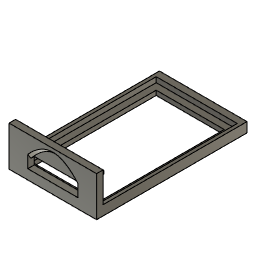
sdr2 (Autodesk Fusion 360 design; units mm, degrees)
Autodesk Fusion 360 part; units mm, degrees
sketch "Sketch1" plane through (0, 0, 0) normal (0, 1, 0) x (1, 0, 0)
  line L0 (0, 0) -> (15, 0)
  line L1 (15, 0) -> (15, -1.85)
  line L2 (15, -1.85) -> (0, -1.85)
  line L3 (0, -1.85) -> (0, 0)
  line L4 (-0.2, -2.05) -> (15.2, -2.05)
  line L5 (15.2, -2.05) -> (15.2, 0.2)
  line L6 (15.2, 0.2) -> (-0.2, 0.2)
  line L7 (-0.2, 0.2) -> (-0.2, -2.05)
  spline S0 degree 5 poles (-0.2, -2.05) (0.108, -2.4292) (0.724, -3.1546) (1.648, -4.1433) (2.88, -5.2595) (4.42, -6.2953) (5.96, -6.9394) (7.5, -7.16) (9.04, -6.9394) (10.58, -6.2953) (12.12, -5.2595) (13.352, -4.1433) (14.276, -3.1546) (14.892, -2.4292) (15.2, -2.05) knots 0 0 0 0 0 0 0.1 0.2 0.3 0.4 0.5 0.6 0.7 0.8 0.9 1 1 1 1 1 1
  line L8 (-6.2, -9.05) -> (21.2, -9.05)
  line L9 (21.2, -9.05) -> (21.2, 3.2)
  line L10 (21.2, 3.2) -> (-6.2, 3.2)
  line L11 (-6.2, 3.2) -> (-6.2, -9.05)
  line L12 (-4.95, 0.2) -> (19.95, 0.2)
  line L13 (19.95, 0.2) -> (19.95, 1.8)
  line L14 (19.95, 1.8) -> (-4.95, 1.8)
  line L15 (-4.95, 1.8) -> (-4.95, 0.2)
  line L16 (-4.95, 0.2) -> (-5.95, 0.2)
  line L17 (-5.95, 0.2) -> (-5.95, 3.2)
  line L18 (-5.95, 3.2) -> (-4.95, 3.2)
  line L19 (-4.95, 3.2) -> (-4.95, 0.2)
  line L20 (19.95, 0.2) -> (20.95, 0.2)
  line L21 (20.95, 0.2) -> (20.95, 3.2)
  line L22 (20.95, 3.2) -> (19.95, 3.2)
  line L23 (19.95, 3.2) -> (19.95, 0.2)
  point P0 (7.5, -7.05)
  dimension "d1" = 15
  dimension "d2" = 1.85
  dimension "d3" = 0.2
  dimension "d4" = 0.2
  dimension "d5" = 0.2
  dimension "d6" = 0.2
  dimension "d8" = 5
  dimension "d9" = 3
  dimension "d10" = 6
  dimension "d11" = 6
  dimension "d12" = 7
  dimension "d13" = 24.9
  dimension "d14" = 1.6
  dimension "d15" = 4.75
  dimension "d24" = 1
  dimension "d25" = 1
  dimension "d26" = 3
  constraint horizontal L0
  constraint vertical L1
  constraint horizontal L2
  constraint vertical L3
  constraint coincident L0.start L3.end
  constraint horizontal L4
  constraint vertical L5
  constraint horizontal L6
  constraint vertical L7
  constraint horizontal L8
  constraint vertical L9
  constraint horizontal L10
  constraint vertical L11
  constraint horizontal L12
  constraint vertical L13
  constraint horizontal L14
  constraint vertical L15
  constraint horizontal L16
  constraint vertical L17
  constraint horizontal L18
  constraint vertical L19
  constraint horizontal L20
  constraint vertical L21
  constraint horizontal L22
  constraint vertical L23
  measures "d1" distance of L0.start L0.end
  measures "d2" distance of L0.start L2.end
  measures "d3" distance of L3 L7
  measures "d4" distance of L2 L4
  measures "d5" distance of L1 L5
  measures "d6" distance of L0 L6
  measures "d8" distance of L4 P0
  measures "d9" distance of L6 L10
  measures "d10" distance of L7 L11
  measures "d11" distance of L5 L9
  measures "d12" distance of L4 L8
  measures "d13" distance of L12.start L12.end
  measures "d14" distance of L12.start L14.end
  measures "d15" distance of L7 L15
  measures "d24" distance of L12.start L16.end
  measures "d25" distance of L12.end L20.end
  measures "d26" distance of L12.end L22.end
extrude "Extrude1" add sketch "Sketch1" against normal blind 2 contours L5 L7 S0 L8 L9 L10 L11 L12 L16 L17 L20 L21 | L10 L15 L16 L17 L18 L19 | L10 L13 L20 L21 L22 L23 | L10 L14 L19 L23
extrude "Extrude2" add sketch "Sketch1" against normal blind 1 contours L4 S0
chamfer "Chamfer1" distance 1 angle 45 1 edges at (7.5, -1, 2.05)
chamfer "Chamfer2" distance 1 angle 45 1 edges at (7.5, -2, 7.05)
extrude "Extrude3" add sketch "Sketch1" against normal blind 2 contours L6 L12 L13 L14 L15 L19 L23
extrude "Extrude4" add sketch "Sketch1" along normal blind 42.2 contours L10 L15 L16 L17 L18 L19 | L10 L13 L20 L21 L22 L23 | L10 L14 L19 L23
sketch "Sketch2" plane through (0, 42.2, 0) normal (0, 1, 0) x (-1, 0, 0)
  line L0 (-19.95, -0.2) -> (-20.95, -0.2)
  line L1 (-20.95, -0.2) -> (-20.95, -3.2)
  line L2 (-20.95, -3.2) -> (5.95, -3.2)
  line L3 (5.95, -3.2) -> (5.95, -0.2)
  line L4 (5.95, -0.2) -> (4.95, -0.2)
  line L5 (4.95, -0.2) -> (4.95, -1.8)
  line L6 (4.95, -1.8) -> (-19.95, -1.8)
  line L7 (-19.95, -1.8) -> (-19.95, -0.2)
  line L8 (-20.95, -0.2) -> (5.95, -0.2)
  line L9 (5.95, -0.2) -> (5.95, -3.2)
  line L10 (5.95, -3.2) -> (-20.95, -3.2)
  line L11 (-20.95, -3.2) -> (-20.95, -0.2)
  constraint horizontal L8
  constraint vertical L9
  constraint horizontal L10
  constraint vertical L11
  constraint coincident L2.end L3.start
  constraint coincident L0.end L1.start
extrude "Extrude5" add sketch "Sketch2" along normal blind 2
sketch "Sketch3" plane through (0, 0, -1.8) normal (0, 0, 1) x (-1, 0, 0)
  line L0 (4.95, 0) -> (-19.95, 0)
  line L1 (-19.95, 0) -> (-19.95, -42.2)
  line L2 (-19.95, -42.2) -> (4.95, -42.2)
  line L3 (4.95, -42.2) -> (4.95, 0)
  line L4 (2.95, -2) -> (-17.95, -2)
  line L5 (-17.95, -2) -> (-17.95, -40.2)
  line L6 (-17.95, -40.2) -> (2.95, -40.2)
  line L7 (2.95, -40.2) -> (2.95, -2)
  line L8 (6.2, 0) -> (-21.2, 0)
  dimension "d31" = 2
  dimension "d32" = 2
  dimension "d33" = 2
  dimension "d34" = 2
  constraint horizontal L4
  constraint vertical L5
  constraint horizontal L6
  constraint vertical L7
  measures "d31" distance of L2 L6
  measures "d32" distance of L1 L5
  measures "d33" distance of L4 L8
  measures "d34" distance of L3 L7
extrude "Extrude6" cut sketch "Sketch3" against normal blind 3 contours L4 L5 L6 L7
extrude "Extrude7" cut 1 faces at (-6.2, -0.6667, 0.8833) along direction (1, 0, 0) blind 0.25
extrude "Extrude8" cut 1 faces at (21.2, -0.6667, 4.9667) along direction (-1, 0, 0) blind 0.25
sketch "Sketch4" plane through (0, 0, 0) normal (0, 1, 0) x (-1, 0, 0)
  line L0 (-20.95, 9.05) -> (-20.95, -0.2)
  line L1 (-20.95, -0.2) -> (-19.95, -0.2)
  line L2 (-19.95, -0.2) -> (-19.95, -1.8)
  line L3 (-19.95, -1.8) -> (4.95, -1.8)
  line L4 (4.95, -1.8) -> (4.95, -0.2)
  line L5 (4.95, -0.2) -> (5.95, -0.2)
  line L6 (5.95, -0.2) -> (5.95, 9.05)
  line L7 (5.95, 9.05) -> (-20.95, 9.05)
  line L8 (-15.2, -0.2) -> (-15.2, 2.05)
  line L9 (-15.2, 2.05) -> (0.2, 2.05)
  line L10 (0.2, 2.05) -> (0.2, -0.2)
  line L11 (0.2, -0.2) -> (-15.2, -0.2)
  line L12 (-15.2, 2.05) -> (0.2, 2.05)
  line L13 (0.2, 2.05) -> (0.2, 6.05)
  line L14 (0.2, 6.05) -> (-15.2, 6.05)
  line L15 (-15.2, 6.05) -> (-15.2, 2.05)
  dimension "d41" = 15.4
  dimension "d42" = 4
  constraint horizontal L12
  constraint vertical L13
  constraint horizontal L14
  constraint vertical L15
  constraint coincident L8.end L9.start
  measures "d41" distance of L8.end L9.end
  measures "d42" distance of L8.end L14.end
extrude "Extrude9" add sketch "Sketch4" along normal blind 6 contours L9 L12 L13 L14 L15
chamfer "Chamfer3" distance 1 angle 75 1 edges at (7.5, 0, 2.05) measured on face at (5.2178, -0.3335, 2.3833)
chamfer "Chamfer4" distance 3 angle 45 1 edges at (7.5, 6, 6.05)
